Untitled (Autodesk Fusion 360 design; units mm, degrees)
Autodesk Fusion 360 part; units mm, degrees
sketch "shape" plane through (0, 0, 0) normal (0, 1, 0) x (1, 0, 0)
  line L0 (170.5738, 28.4165) -> (-42.7862, 28.4165)
  line L1 (-42.7862, 28.4165) -> (-42.7862, -100.0835)
  line L2 (170.5738, -100.0835) -> (170.5738, 28.4165)
  line L3 (-42.7862, -100.0835) -> (170.5738, -100.0835)
  line L4 (-42.7862, 28.4165) -> (-42.7862, 29.4165)
  line L5 (-42.7862, 28.4165) -> (-43.7862, 28.4165)
  line L6 (-42.7862, 28.4165) -> (-43.7862, 28.4165)
  line L7 (-43.7862, 28.4165) -> (-43.7862, 29.4165)
  line L8 (-43.7862, 29.4165) -> (-42.7862, 29.4165)
  line L9 (-42.7862, 29.4165) -> (-42.7862, 28.4165)
  line L10 (-43.7862, 29.4165) -> (171.5738, 29.4165)
  line L11 (171.5738, 29.4165) -> (171.5738, -101.0835)
  line L12 (171.5738, -101.0835) -> (-43.7862, -101.0835)
  line L13 (-43.7862, -101.0835) -> (-43.7862, 29.4165)
  dimension "d1" = 213.36
  dimension "d2" = 128.5
  dimension "d3" = 1
  dimension "d4" = 1
  dimension "d5" = 130.5
  constraint perpendicular L0 L4
  constraint horizontal L6
  constraint vertical L7
  constraint horizontal L8
  constraint vertical L9
  constraint horizontal L10
  constraint vertical L11
  constraint horizontal L12
  constraint vertical L13
  measures "d1" distance of L1 L2
  measures "d2" distance of L0 L3
  measures "d3" distance of L0.end L4.end
  measures "d4" distance of L0.end L5.end
  measures "d5" distance of L7.end L12.end
extrude "Extrude1" add sketch "shape" along normal blind 1 contours L0 L1 L2 L3
extrude "Extrude2" add sketch "shape" along normal blind 106
